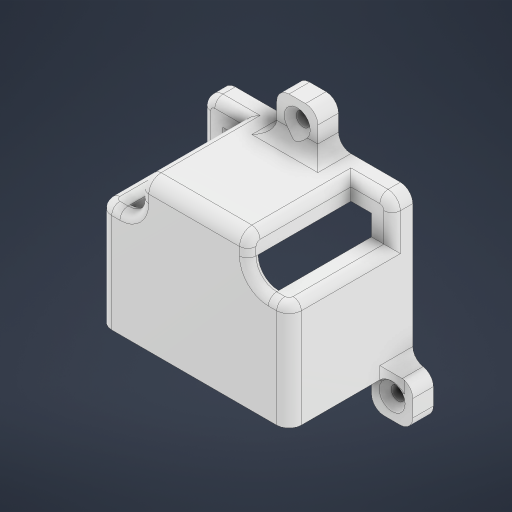
# Autodesk Inventor part: BackBracket
Saved by Autodesk Inventor 2023 (Build 270158000, 158)
## iProperties
Created: 2023-09-27
Part Number: BackBracket
Material: Пластик ПАЭК
Document SubType Name: Modeling
Designer: khrip
Density: 1.32 g/cm^3
Appearance: Гладкий — белый
Author: khrip
Autodesk Inventor part; units mm, degrees
ref_plane "YZ Plane" through (0, 0, 0) normal (1, 0, 0) x (0, 1, 0)
ref_plane "РабПлоскость1" through (0, 0, 0) normal (0, 0, 1) x (1, 0, 0)
sketch "Эскиз1" plane through (0, 0, 0) normal (0, 0, 1) x (1, 0, 0)
  line L0 (-36, -50.525) -> (-10, -50.525)
  line L1 (-10, -50.525) -> (-10, 46.475)
  line L2 (-10, 46.475) -> (-36, 46.475)
  line L3 (-36, 46.475) -> (-36, -50.525)
  line L4 (-40, 46.475) -> (-40, -50.525) projected
  line L5 (-41, -55.525) -> (-5, -55.525)
  line L6 (-5, -55.525) -> (-5, 51.475)
  line L7 (-5, 51.475) -> (-41, 51.475)
  line L8 (-41, 51.475) -> (-41, -55.525)
  line L9 (-36, 51.475) -> (-10, 51.475)
  line L10 (-10, 51.475) -> (-10, 56.475)
  line L11 (-10, 56.475) -> (-36, 56.475)
  line L12 (-36, 56.475) -> (-36, 51.475)
  line L13 (-5, 46.475) -> (0, 46.475)
  line L14 (0, 46.475) -> (0, 20.475)
  line L15 (0, 20.475) -> (-5, 20.475)
  line L16 (-5, 20.475) -> (-5, 46.475)
  line L17 (-41, 46.475) -> (-46, 46.475)
  line L18 (-46, 46.475) -> (-46, 20.475)
  line L19 (-46, 20.475) -> (-41, 20.475)
  line L20 (-41, 20.475) -> (-41, 46.475)
  line L21 (-10, 50.475) -> (-36, 50.475) projected
  point P0 (0, 0)
  dimension "d0" = 1
  dimension "d1" = 5
  dimension "d2" = 26
  dimension "d3" = 5
  dimension "d4" = 26
  dimension "d5" = 5
  dimension "d6" = 5
  dimension "d7" = 5
  dimension "d8" = 1
  constraints: 40 end point, 6 parallel, 5 horizontal, 4 point on line, 3 perpendicular, 2 vertical, 7 other
  measures "d0" distance between parallel lines of L4 L8
  measures "d1" distance of L10.end L9.end
  measures "d2" distance between parallel lines of L12 L10
  measures "d3" distance of L14.end L15.end
  measures "d4" distance of L13.end L14.end
  measures "d5" distance between parallel lines of L7 L13
  measures "d6" distance of L19.end L18.end
  measures "d7" distance between parallel lines of L17 L7
  measures "d8" distance between parallel lines of L9 L21
ref_plane "РабПлоскость2" through (-36, -50.525, 27) normal (0, 0, 1) x (1, 0, 0)
extrude "Выдавливание1" add sketch "Эскиз1" along normal blind 27.5 contours L19 L18 L17 L8 | L6 L13 L14 L15 | L12 L11 L10 L7
sketch "Эскиз2" plane through (0, 0, 0) normal (0, 0, 1) x (1, 0, 0)
  line L0 (-54, 53.525) -> (-54, 61.271) projected
  line L1 (-54, 53.525) -> (-54, -71.6155)
  line L2 (-46, 20.475) -> (-41, 20.475) projected
  line L3 (-41, 20.475) -> (-51, 20.475)
  line L4 (-51, 20.475) -> (-51, 10.475)
  line L5 (-51, 10.475) -> (-41, 10.475)
  line L6 (-41, 10.475) -> (-41, 20.475)
  line L7 (-5, 46.475) -> (-5, 20.475) projected
  line L8 (-5, 20.475) -> (5, 20.475)
  line L9 (5, 20.475) -> (5, 10.475)
  line L10 (5, 10.475) -> (-5, 10.475)
  line L11 (-5, 10.475) -> (-5, 20.475)
  line L12 (-10, 56.475) -> (-36, 56.475) projected
  line L13 (-23, 56.475) -> (-18, 56.475)
  line L14 (-18, 56.475) -> (-18, 66.475)
  line L15 (-18, 66.475) -> (-23, 66.475)
  line L16 (-23, 66.475) -> (-23, 56.475)
  line L17 (-23, 66.475) -> (-28, 66.475)
  line L18 (-28, 66.475) -> (-28, 56.475)
  line L19 (-28, 56.475) -> (-23, 56.475)
  line L20 (-23, 56.475) -> (-23, 66.475)
  line L21 (0, 46.475) -> (-5, 46.475) projected
  line L22 (-5, 46.475) -> (-5, 20.475) projected
  line L23 (-5, 20.475) -> (0, 20.475) projected
  line L24 (0, 20.475) -> (0, 46.475) projected
  line L25 (-36, 56.475) -> (-36, 51.475) projected
  line L26 (-36, 51.475) -> (-10, 51.475) projected
  line L27 (-10, 51.475) -> (-10, 56.475) projected
  line L28 (-10, 56.475) -> (-36, 56.475) projected
  line L29 (-46, 20.475) -> (-41, 20.475) projected
  line L30 (-41, 20.475) -> (-41, 46.475) projected
  line L31 (-41, 46.475) -> (-46, 46.475) projected
  line L32 (-46, 46.475) -> (-46, 20.475) projected
  line L33 (-10, 51.475) -> (0, 51.475)
  line L34 (0, 51.475) -> (0, 56.475)
  line L35 (0, 56.475) -> (-10, 56.475)
  line L36 (-10, 56.475) -> (-10, 51.475)
  line L37 (-5, 46.475) -> (0, 46.475)
  line L38 (0, 46.475) -> (0, 51.475)
  line L39 (0, 51.475) -> (-5, 51.475)
  line L40 (-5, 51.475) -> (-5, 46.475)
  line L41 (-36, 51.475) -> (-46, 51.475)
  line L42 (-46, 51.475) -> (-46, 56.475)
  line L43 (-46, 56.475) -> (-36, 56.475)
  line L44 (-36, 56.475) -> (-36, 51.475)
  line L45 (-46, 51.475) -> (-41, 51.475)
  line L46 (-41, 51.475) -> (-41, 46.475)
  line L47 (-41, 46.475) -> (-46, 46.475)
  line L48 (-46, 46.475) -> (-46, 51.475)
  point P0 (0, 0)
  dimension "d11" = 10
  dimension "d12" = 10
  dimension "d13" = 10
  dimension "d14" = 10
  dimension "d15" = 5
  dimension "d16" = 10
  dimension "d17" = 5
  dimension "d22" = 0
  dimension "d23" = 46
  dimension "d24" = 36
  dimension "d25" = 10
  dimension "d26" = 18
  dimension "d27" = 26
  dimension "d28" = 46
  dimension "d29" = 118.0905
  constraints: 66 end point, 16 parallel, 8 horizontal, 8 perpendicular, 2 point on line, 1 midpoint, 1 vertical
  measures "d11" distance of L5.end L4.end
  measures "d12" distance of L4.end L3.end
  measures "d13" distance of L9.end L10.end
  measures "d14" distance of L8.end L9.end
  measures "d15" distance of L15.end L14.end
  measures "d16" distance of L14.end L13.end
  measures "d17" distance of L19.end L18.end
  measures "d22" distance between parallel lines of L24 L34
  measures "d23" distance between parallel lines of L24 L42
  measures "d24" distance between parallel lines of L23 L35
  measures "d25" distance from line of point (-18, 56.475) L21
  measures "d26" distance from line of point (-18, 56.475) L24
  measures "d27" distance from line of point (-46, 20.475) L21
  measures "d28" distance from line of point (-46, 20.475) L24
  measures "d29" distance from line of L1.end L21
extrude "Выдавливание2" add sketch "Эскиз2" along normal blind 5 contours L2 L6 L5 L4 L3 | L48 L41 L46 L31 | L42 L43 L25 L41 | L27 L35 L34 L33 | L18 L17 L16 L12 | L33 L38 L21 L40 | L16 L15 L14 L12 | L8 L9 L10 L11
sketch "Эскиз3" plane through (0, 0, 27.5) normal (0, 0, 1) x (1, 0, 0)
  line L0 (-46, 46.475) -> (-46, 20.475) projected
  line L1 (-5, 20.475) -> (0, 20.475) projected
  line L2 (-46, 46.475) -> (0, 46.475)
  line L3 (0, 46.475) -> (0, 20.475)
  line L4 (0, 20.475) -> (-46, 20.475)
  line L5 (-46, 20.475) -> (-46, 46.475)
  line L6 (-36, 56.475) -> (-36, 51.475) projected
  line L7 (-36, 51.475) -> (-10, 51.475) projected
  line L8 (-10, 51.475) -> (-10, 56.475) projected
  line L9 (-10, 56.475) -> (-36, 56.475) projected
  line L10 (-36, 56.475) -> (-36, 51.475) projected
  line L11 (-36, 56.475) -> (-10, 56.475)
  line L12 (-10, 56.475) -> (-10, 46.475)
  line L13 (-10, 46.475) -> (-36, 46.475)
  line L14 (-36, 46.475) -> (-36, 56.475)
  point P0 (0, 0)
  constraints: 16 end point, 4 parallel, 2 horizontal, 2 perpendicular, 1 point on line
extrude "Выдавливание3" add sketch "Эскиз3" along normal blind 2.5
sketch "Эскиз4" plane through (0, 0, 5) normal (0, 0, 1) x (1, 0, 0)
  line L0 (-5, 46.475) -> (0, 46.475) projected
  line L1 (0, 56.475) -> (0, 46.475) projected
  line L2 (-10, 56.475) -> (0, 56.475) projected
  line L3 (-18, 56.475) -> (-10, 56.475) projected
  line L4 (-28, 56.475) -> (-18, 56.475) projected
  line L5 (-36, 56.475) -> (-28, 56.475) projected
  line L6 (-46, 56.475) -> (-36, 56.475) projected
  line L7 (-46, 46.475) -> (-46, 56.475) projected
  line L8 (-46, 46.475) -> (-41, 46.475) projected
  line L9 (-41, 51.475) -> (-41, 46.475) projected
  line L10 (-36, 51.475) -> (-41, 51.475) projected
  line L11 (-36, 51.475) -> (-36, 56.475) projected
  line L12 (-5, 46.475) -> (-5, 51.475) projected
  line L13 (-5, 20.475) -> (-5, 46.475) projected
  line L14 (0, 20.475) -> (-5, 20.475) projected
  line L15 (0, 46.475) -> (0, 20.475) projected
  line L16 (-10, 56.475) -> (-10, 51.475) projected
  line L17 (-5, 51.475) -> (-10, 51.475) projected
  line L18 (-18, 66.475) -> (-18, 56.475) projected
  line L19 (-28, 66.475) -> (-18, 66.475) projected
  line L20 (-28, 56.475) -> (-28, 66.475) projected
  line L21 (-46, 20.475) -> (-46, 46.475) projected
  line L22 (-41, 20.475) -> (-46, 20.475) projected
  line L23 (-41, 20.475) -> (-41, 10.475) projected
  line L24 (-41, 10.475) -> (-51, 10.475) projected
  line L25 (-51, 10.475) -> (-51, 20.475) projected
  line L26 (-51, 20.475) -> (-46, 20.475) projected
  line L27 (-41, 46.475) -> (-41, 20.475) projected
  line L28 (-10, 51.475) -> (-36, 51.475) projected
  line L29 (-5, 10.475) -> (-5, 20.475) projected
  line L30 (5, 10.475) -> (-5, 10.475) projected
  line L31 (5, 20.475) -> (5, 10.475) projected
  line L32 (0, 20.475) -> (5, 20.475) projected
  circle A0 centre (0, 15.475) radius 2.1478
  circle A1 centre (-46, 15.475) radius 2.1478
  circle A2 centre (-23, 61.475) radius 2.0368
  point P0 (0, 0)
  constraints: 3 centre point
hole "Отверстие1" at (0, 15.475, 5) at (-46, 15.475, 5) at (-23, 61.475, 5) direction (0, 0, -1) diameter 3.4 end through all countersink diameter 6.3 countersink angle 90 clearance for "Винт с потайной головкой ISO 2009/7046" size "M3" standard "ISO"
fillet "Сопряжение1" radius 3 17 edges at (0, 20.475, 2.5) (0, 56.475, 2.5) (-46, 20.475, 2.5) (-46, 56.475, 2.5) (-28, 56.475, 2.5) (-18, 56.475, 2.5) (-28, 66.475, 2.5) (-18, 66.475, 2.5) (-51, 20.475, 2.5) (-51, 10.475, 2.5) (-41, 10.475, 2.5) (-5, 10.475, 2.5) (5, 10.475, 2.5) (5, 20.475, 2.5) (-46, 33.475, 30) (0, 33.475, 30) (-23, 56.475, 30)
fillet "Сопряжение2" radius 5 2 edges at (-36, 46.475, 28.75) (-10, 46.475, 28.75)
fillet "Сопряжение3" radius 2 20 edges at (-0.8787, 55.5963, 5) (-6.5, 56.475, 5) (0, 49.975, 5) (-4, 46.475, 30) (-0.8787, 46.475, 29.1213) (0, 46.475, 16) (-10, 52.475, 30) (-10, 55.5963, 29.1213) (-10, 56.475, 16) (-8.5355, 47.9395, 30) (-37.4645, 47.9395, 30) (-42, 46.475, 30) (-45.1213, 46.475, 29.1213) (-46, 46.475, 16) (-36, 55.5963, 29.1213) (-36, 56.475, 16) (-36, 52.475, 30) (-45.1213, 55.5963, 5) (-39.5, 56.475, 5) (-46, 49.975, 5)
fillet "Сопряжение4" radius 3 7 edges at (0, 21.975, 5) (-2.5, 20.475, 5) (-43.5, 20.475, 5) (-46, 21.975, 5) (-29.5, 56.475, 5) (-23, 56.475, 5) (-16.5, 56.475, 5)
